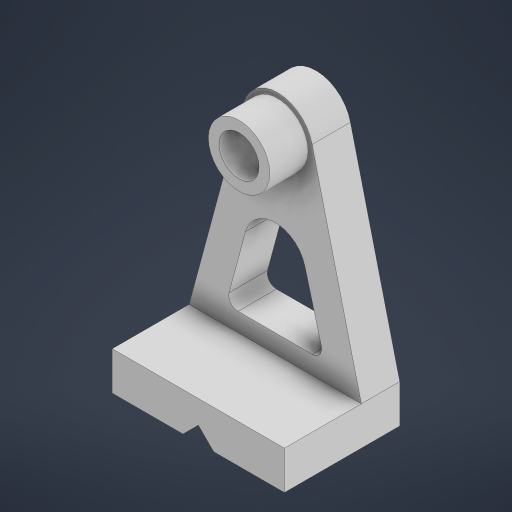
# Autodesk Inventor part: Część2
Saved by Autodesk Inventor 2023 (Build 270158000, 158)
## iProperties
Created: 2023-05-07
Part Number: Część2
Material: Ogólny
Document SubType Name: Modeling
Designer: Adam
Density: 1 g/cm^3
Appearance: Domyślna
Author: Adam
Autodesk Inventor part; units mm, degrees
ref_plane "YZ Plane" through (0, 0, 0) normal (1, 0, 0) x (0, 1, 0)
ref_plane "XZ Plane" through (0, 0, 0) normal (0, 1, 0) x (-1, 0, 0)
ref_plane "XY Plane" through (0, 0, 0) normal (0, 0, 1) x (1, 0, 0)
sketch "Szkic1" plane through (0, 0, 0) normal (0, 1, 0) x (-1, 0, 0)
  line L0 (56, -37.5) -> (-56, -37.5)
  line L1 (-56, -37.5) -> (-56, 37.5)
  line L2 (-56, 37.5) -> (56, 37.5)
  line L3 (56, 37.5) -> (56, -37.5)
  line L4 (56, -37.5) -> (-56, 37.5) construction
  line L5 (-56, -37.5) -> (56, 37.5) construction
  point P0 (0, 0)
  dimension "d0" = 112
  dimension "d1" = 75
  constraints: 12 end point, 2 midpoint, 2 parallel, 1 horizontal, 1 perpendicular
  measures "d0" distance of L1.end L2.end
  measures "d1" distance of L0.end L1.end
extrude "Wyciągnięcie proste1" add sketch "Szkic1" along normal blind 25
sketch "Szkic2" plane through (0, 25, 0) normal (0, 1, 0) x (1, 0, 0)
  line L0 (56, 37.5) -> (-56, 37.5) projected
  line L1 (56, -37.5) -> (56, 37.5) projected
  line L2 (-56, 37.5) -> (56, 37.5)
  line L3 (56, 37.5) -> (56, 12.5)
  line L4 (56, 12.5) -> (-56, 12.5)
  line L5 (-56, 12.5) -> (-56, 37.5)
  point P0 (0, 0)
  dimension "d4" = 25
  constraints: 8 end point, 2 parallel, 1 horizontal, 1 perpendicular, 1 point on line
  measures "d4" distance between parallel lines of L4 L0
extrude "Wyciągnięcie proste2" add sketch "Szkic2" along normal blind 148
sketch "Szkic3" plane through (-56, 25, -12.5) normal (0, 0, 1) x (1, 0, 0)
  circle A0 centre (57.4852, 125) radius 23
  line L0 (0, 0) -> (112, 0) projected
  line L1 (112, -25) -> (112, 148) projected
  line L2 (0, -25) -> (0, 148) projected
  line L3 (0, 0) -> (0, 148)
  line L4 (0, 148) -> (112, 148) projected
  line L5 (0, 148) -> (112, 148)
  line L6 (112, 148) -> (112, 0)
  line L7 (0, 0) -> (35.2766, 130.9813)
  line L8 (79.6938, 130.9813) -> (112, 0)
  point P0 (56, -25)
  point P1 (79.928, 130.0318)
  point P2 (57.4852, 148)
  dimension "d8" = 46
  constraints: 10 end point, 2 collinear, 2 point on circle, 1 centre point, 1 perpendicular, 1 point on line, 1 tangent
  measures "d8" diameter of A0
extrude "Wyciągnięcie proste3" cut sketch "Szkic3" against normal blind 25 contours L7 L2 L4 A0 | L4 L1 L8 A0
sketch "Szkic4" plane through (-56, 25, -12.5) normal (0, 0, 1) x (1, 0, 0)
  arc A0 (79.928, 130.0318) -> (35.2766, 130.9813) centre (57.4852, 125) ccw projected
  circle A1 centre (57.4852, 125) radius 20
  point P0 (56, -25)
  dimension "d11" = 40
  constraints: 2 coincident, 1 centre point
  measures "d11" diameter of A1
extrude "Wyciągnięcie proste4" add sketch "Szkic4" along normal blind 25
sketch "Szkic5" plane through (-56, 25, -12.5) normal (0, 0, 1) x (1, 0, 0)
  line L0 (56, 12) -> (31.7743, 12)
  line L1 (25.9808, 19.5604) -> (42.2104, 79.8208)
  line L2 (0, 0) -> (112, 0) projected
  line L3 (35.2766, 130.9813) -> (0, 0) projected
  arc A0 (25.9808, 19.5604) -> (31.7743, 12) centre (31.7743, 18) ccw
  circle A1 centre (57.4852, 125) radius 20 projected
  line L4 (56, 12) -> (80.2257, 12)
  line L5 (86.0192, 19.5604) -> (69.7896, 79.8208)
  arc A2 (80.2257, 12) -> (86.0192, 19.5604) centre (80.2257, 18) ccw
  circle A3 centre (56, 54.1155) radius 20
  point P0 (56, -25)
  point P1 (75.3119, 59.3167)
  point P2 (36.6881, 59.3167)
  dimension "d14" = 12
  dimension "d15" = 20
  dimension "d16" = 6
  dimension "d17" = 40
  constraints: 8 end point, 4 point on circle, 3 centre point, 3 tangent, 1 horizontal, 1 parallel
  measures "d14" distance between parallel lines of L2 L0
  measures "d15" distance between parallel lines of L1 L3
  measures "d16" radius of A0
  measures "d17" diameter of A3
extrude "Wyciągnięcie proste5" cut sketch "Szkic5" against normal blind 25 contours L0 A0 L1 A3 L5 A2 L4 | A3
sketch "Szkic6" plane through (1.4852, 150, 12.5) normal (0, 0, 1) x (1, 0, 0)
  point P0 (-1.4852, -150)
  point P1 (0, 0)
hole "Otwór1" at (1.4852, 150, 12.5) direction (0, 0, -1) diameter 26 end through all
sketch "Szkic7" plane through (0, 0, 0) normal (0, -1, 0) x (1, 0, 0)
  point P0 (0, 0)
sketch "Szkic8" plane through (-56, 0, 37.5) normal (0, 0, 1) x (1, 0, 0)
  line L0 (112, 0) -> (0, 0) projected
  line L1 (46, 0) -> (66, 0)
  line L2 (0, 0) -> (112, 0) projected
  line L3 (46, 0) -> (56, 10)
  line L4 (46, 0) -> (60.1421, 0) construction
  line L5 (56, 10) -> (66, 0)
  point P0 (56, 0)
  dimension "d27" = 20
  dimension "d28" = 45
  constraints: 8 end point, 1 collinear, 1 equal length, 1 horizontal, 1 perpendicular, 1 point on line
  measures "d27" distance of L1.start L1.end
  measures "d28" angle of L4 L3
extrude "Wyciągnięcie proste6" cut sketch "Szkic8" against normal blind 75
